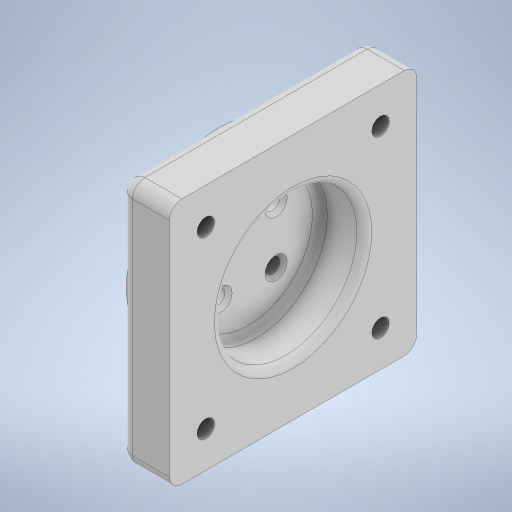
# Autodesk Inventor part: adaptador para abb
Saved by Autodesk Inventor 2024 (Build 280153000, 153)
## iProperties
Created: 2026-04-16
Part Number: adaptador para abb
Material: Genérico
Document SubType Name: Modeling
Designer: Legion
Density: 1 g/cm^3
Appearance: Valor por defecto
Author: Legion
Autodesk Inventor part; units mm, degrees
ref_plane "YZ Plane" through (0, 0, 0) normal (1, 0, 0) x (0, 1, 0)
ref_plane "XZ Plane" through (0, 0, 0) normal (0, 1, 0) x (-1, 0, 0)
ref_plane "XY Plane" through (0, 0, 0) normal (0, 0, 1) x (1, 0, 0)
sketch "Boceto1" plane through (0, 0, 0) normal (1, 0, 0) x (0, 1, 0)
  circle A0 centre (0, 0) radius 37.5
  circle A1 centre (0, 0) radius 20.2
  line L0 (0, 0) -> (50, 0)
  line L1 (0, 0) -> (-50, 0)
  line L2 (0, 0) -> (0, -50)
  line L3 (0, 0) -> (0, 50)
  dimension "d0" = 75
  dimension "d1" = 40.4
  dimension "d2" = 50
  dimension "d3" = 50
  dimension "d4" = 50
  dimension "d5" = 50
  constraints: 8 end point, 2 centre point, 2 coincident, 2 horizontal, 2 vertical
  measures "d0" diameter of A0
  measures "d1" diameter of A1
  measures "d2" distance of L0.start L0.end
  measures "d3" distance of L0.start L1.end
  measures "d4" distance of L0.start L2.end
  measures "d5" distance of L0.start L3.end
extrude "Extrusión1" add sketch "Boceto1" against normal blind 5 contours L0 L3 A1 | A1 L2 L0 | L3 L1 A1 | A1 L1 L2
extrude "Extrusión2" add sketch "Boceto1" against normal blind 10 contours L0 A1 L3 A0 | A0 L2 A1 L0 | L3 A1 L1 A0 | A0 L1 A1 L2
sketch "Boceto2" plane through (0, 0, 0) normal (1, 0, 0) x (0, 0, -1)
  line L0 (0, 0) -> (0, 50)
  line L1 (0, 0) -> (0, -50)
  line L2 (0, 0) -> (50, 0)
  line L3 (0, 0) -> (-50, 0)
  line L4 (-50, 50) -> (50, 50)
  line L5 (50, 50) -> (50, -50)
  line L6 (50, -50) -> (-50, -50)
  line L7 (-50, -50) -> (-50, 50)
  dimension "d10" = 50
  dimension "d11" = 50
  dimension "d12" = 50
  dimension "d13" = 50
  constraints: 16 end point, 3 horizontal, 2 parallel, 2 vertical, 1 perpendicular
  measures "d10" distance of L0.start L0.end
  measures "d11" distance of L0.start L1.end
  measures "d12" distance of L0.start L2.end
  measures "d13" distance of L0.start L3.end
extrude "Extrusión3" add sketch "Boceto2" along normal blind 20
sketch "Boceto3" plane through (20, 0, 0) normal (1, 0, 0) x (0, 0, -1)
  circle A0 centre (0, 0) radius 37.5 projected
  circle A1 centre (0, 0) radius 20.2 projected
  circle A2 centre (0, 0) radius 20.2 projected
  line L0 (0, 20.2) -> (0, 37.5)
  circle A3 centre (0, 0) radius 28.85
  circle A4 centre (0, 0) radius 15.75
  line L1 (-11.1369, -11.1369) -> (11.1369, 11.1369)
  line L2 (0, 0) -> (15.75, 0) construction
  line L3 (11.1369, -11.1369) -> (-11.1369, 11.1369)
  point P0 (0, 15.75)
  dimension "d16" = 31.5
  dimension "d17" = 45
  constraints: 8 end point, 6 coincident, 5 point on circle, 2 centre point, 2 midpoint, 2 vertical alignment, 1 horizontal, 1 vertical, 2 other
  measures "d16" diameter of A4
  measures "d17" angle of L2 L1
extrude "Extrusión4" cut sketch "Boceto3" against normal blind 18 contours A1 | A3 | A4 L3 L1 | L1 L3 A4 | A4 L1 L3 | L3 L1 A4
sketch "Boceto4" plane through (2, 0, 0) normal (1, 0, 0) x (0, 0, -1)
  point P0 (0, 0)
  point P1 (11.1369, -11.1369)
  point P2 (-11.1369, -11.1369)
  point P3 (-11.1369, 11.1369)
  point P4 (11.1369, 11.1369)
hole "Agujero1" at (2, -11.1369, -11.1369) at (2, -11.1369, 11.1369) at (2, 11.1369, 11.1369) at (2, 11.1369, -11.1369) direction (-1, 0, 0) diameter 6 end through all countersink diameter 9 countersink angle 90
sketch "Boceto5" plane through (20, 0, 0) normal (1, 0, 0) x (0, 0, -1)
  circle A0 centre (0, 0) radius 50
  line L0 (-50, -50) -> (50, -50) projected
  line L1 (-35.3553, 35.3553) -> (50, -50)
  line L2 (50, -50) -> (0, 0)
  line L3 (-50, -50) -> (35.3553, 35.3553)
  point P0 (35.3553, -35.3553)
  point P1 (-35.3553, -35.3553)
  constraints: 6 end point, 4 point on circle, 4 point on line, 3 coincident, 1 centre point, 1 collinear, 1 perpendicular
hole "Agujero2" at (20, -35.3553, -35.3553) at (20, -35.3553, 35.3553) at (20, 35.3553, 35.3553) at (20, 35.3553, -35.3553) direction (-1, 0, 0) diameter 7 end through all
sketch "Boceto6" plane through (0, 0, 0) normal (-1, 0, 0) x (0, 0, 1)
  circle A0 centre (-35.3553, 35.3553) radius 3.5
  line L0 (-39.3391, 37.6553) -> (-35.3553, 39.9553)
  line L1 (-35.3553, 39.9553) -> (-31.3716, 37.6553)
  line L2 (-31.3716, 37.6553) -> (-31.3716, 33.0553)
  line L3 (-31.3716, 33.0553) -> (-35.3553, 30.7553)
  line L4 (-35.3553, 30.7553) -> (-39.3391, 33.0553)
  line L5 (-39.3391, 33.0553) -> (-39.3391, 37.6553)
  line L6 (-35.3553, 35.3553) -> (-35.3553, 39.9553)
  circle A1 centre (35.3553, 35.3553) radius 3.5
  circle A2 centre (35.3553, -35.3553) radius 3.5
  circle A3 centre (-35.3068, -35.4038) radius 3.5
  line L7 (31.3716, 37.6553) -> (35.3553, 39.9553)
  line L8 (31.3716, 33.0553) -> (31.3716, 37.6553)
  line L9 (35.3553, 30.7553) -> (31.3716, 33.0553)
  line L10 (39.3391, 33.0553) -> (35.3553, 30.7553)
  line L11 (39.3391, 37.6553) -> (39.3391, 33.0553)
  line L12 (35.3553, 39.9553) -> (39.3391, 37.6553)
  line L13 (31.3716, -33.0553) -> (35.3553, -30.7553)
  line L14 (31.3716, -37.6553) -> (31.3716, -33.0553)
  line L15 (35.3553, -39.9553) -> (31.3716, -37.6553)
  line L16 (39.3391, -37.6553) -> (35.3553, -39.9553)
  line L17 (39.3391, -33.0553) -> (39.3391, -37.6553)
  line L18 (35.3553, -30.7553) -> (39.3391, -33.0553)
  line L19 (-39.3391, -33.1038) -> (-35.3553, -30.8038)
  line L20 (-39.3391, -37.7038) -> (-39.3391, -33.1038)
  line L21 (-35.3553, -40.0038) -> (-39.3391, -37.7038)
  line L22 (-31.3716, -37.7038) -> (-35.3553, -40.0038)
  line L23 (-31.3716, -33.1038) -> (-31.3716, -37.7038)
  line L24 (-35.3553, -30.8038) -> (-31.3716, -33.1038)
  line L25 (-35.3553, -35.4038) -> (-35.3553, -30.8038)
  circle A4 centre (35.3553, -35.3553) radius 3.5 projected
  point P0 (0, 0)
  point P1 (-50, 50)
  constraints: 52 end point, 12 parallel, 6 vertical, 4 centre point
extrude "Extrusión5" cut sketch "Boceto6" against normal blind 6 contours A0 | L0 L1 L2 L3 L4 L5 | A1 | A2 | A3 | L7 L12 L11 L10 L9 L8 | L13 L18 L17 L16 L15 L14 | L19 L24 L23 L22 L21 L20
fillet "Empalme1" radius 1 2 edges at (-5, -20.2, 0) (-10, -20.2, 0)
fillet "Empalme2" radius 3 1 edges at (0, -37.5, 0)
fillet "Empalme3" radius 5 8 edges at (10, -50, 50) (10, -50, -50) (0, -50, 0) (0, 0, 50) (10, 50, 50) (0, 50, 0) (0, 0, -50) (10, 50, -50)
fillet "Empalme4" radius 3 2 edges at (2, 0, 28.85) (20, 0, 28.85)
